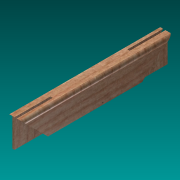
# Autodesk Inventor part: Stretcher-08
Saved by Autodesk Inventor 2013 (Build 170138000, 138)
## iProperties
Created: 2013-08-15
Part Number: Stretcher-08
Material: Wood (Birch)
Document SubType Name: Modeling
Designer: Sawaiz
Density: 1 g/cm^3
Author: Sawaiz
Autodesk Inventor part; units mm, degrees
ref_plane "YZ Plane" through (0, 0, 0) normal (1, 0, 0) x (0, 1, 0)
ref_plane "XZ Plane" through (0, 0, 0) normal (0, 1, 0) x (-1, 0, 0)
ref_plane "XY Plane" through (0, 0, 0) normal (0, 0, 1) x (1, 0, 0)
sketch "Sketch1" plane through (0, 0, 0) normal (1, 0, 0) x (0, 1, 0)
  line L0 (-19.05, 6.858) -> (19.05, 6.858)
  line L1 (19.05, 6.858) -> (19.05, -6.858)
  line L2 (19.05, -6.858) -> (-19.05, -6.858)
  line L3 (-19.05, -6.858) -> (-19.05, 6.858)
  line L4 (-19.05, 6.858) -> (19.05, -6.858) construction
  line L5 (19.05, 6.858) -> (-19.05, -6.858) construction
  arc A0 (19.05, 6.858) -> (10.414, 6.858) centre (14.732, 4.0649) ccw
  arc A1 (10.414, -6.858) -> (19.05, -6.858) centre (14.732, -4.0649) ccw
  line L6 (14.732, 9.2075) -> (14.732, -9.2075)
  point P0 (0, 0)
  dimension "d0" = 38.1
  dimension "d1" = 13.716
  dimension "d6" = 8.636
  dimension "d8" = 8.636
  dimension "d9" = 18.415
  constraints: 14 end point, 6 point on circle, 2 centre point, 2 midpoint, 2 parallel, 2 point on line, 1 equal radius, 1 horizontal, 1 perpendicular
  measures "d0" distance of L1.end L2.end
  measures "d1" distance of L0.end L1.end
  measures "d6" distance of A0.end L0.end
  measures "d8" distance of A1.start L1.end
  measures "d9" distance of L6.start L6.end
extrude "Extrusion1" add sketch "Sketch1" along normal mid plane 203.2
sketch "Sketch3" plane through (-101.6, -19.05, -6.858) normal (0, -1, 0) x (1, 0, 0)
  line L0 (0, 0) -> (203.2, 0) projected
  line L1 (203.2, 13.716) -> (203.2, 0) projected
  line L2 (203.2, 13.716) -> (0, 13.716) projected
  line L3 (0, 0) -> (0, 13.716) projected
  line L4 (203.2, 6.858) -> (154.94, 6.858)
  line L5 (154.94, 6.858) -> (154.94, 3.8)
  line L6 (154.94, 3.8) -> (203.2, 3.8)
  line L7 (203.2, 3.8) -> (203.2, 6.858)
  line L8 (154.94, 6.858) -> (203.2, 6.858)
  line L9 (203.2, 6.858) -> (203.2, 9.916)
  line L10 (0, 9.916) -> (48.26, 9.916)
  line L11 (48.26, 9.916) -> (48.26, 6.858)
  line L12 (48.26, 6.858) -> (0, 6.858)
  line L13 (0, 6.858) -> (0, 9.916)
  point P0 (101.6, 6.858)
  dimension "d14" = 48.26
  dimension "d19" = 3.8
  dimension "d21" = 3.058
  dimension "d22" = 48.26
  dimension "d23" = 3.8
  dimension "d24" = 3.058
  constraints: 20 end point, 4 parallel, 3 horizontal, 3 perpendicular, 2 point on line, 1 midpoint
  measures "d14" distance between parallel lines of L7 L5
  measures "d19" distance between parallel lines of L0 L6
  measures "d21" distance of L4.end L5.end
  measures "d22" distance between parallel lines of L11 L13
  measures "d23" distance between parallel lines of L2 L10
  measures "d24" distance between parallel lines of L12 L10
extrude "Extrusion3" cut sketch "Sketch3" against normal through all contours L3 L10 L11 L12 | L6 L5 L4 L1
ref_plane "Work Plane1" through (-101.6, 10.414, 26.858) normal (0, 0, 1) x (1, 0, 0)
sketch "Sketch4" plane through (-101.6, 10.414, 26.858) normal (0, 0, 1) x (1, 0, 0)
  line L0 (0, 0) -> (203.2, 0) projected
  line L1 (0, -29.464) -> (0, 0) projected
  line L2 (203.2, -29.464) -> (0, -29.464) projected
  line L3 (203.2, 0) -> (203.2, -29.464) projected
  line L4 (0, 0) -> (203.2, 0) projected
  line L5 (203.2, 8.636) -> (203.2, 0) projected
  line L6 (0, 8.636) -> (203.2, 8.636) projected
  line L7 (0, 0) -> (0, 8.636) projected
  line L8 (203.2, 8.636) -> (165.1, -29.464)
  line L9 (0, 8.636) -> (38.1, -29.464)
  line L10 (203.2, 8.636) -> (203.2, -29.464)
  line L11 (165.1, -29.464) -> (203.2, -29.464)
  line L12 (38.1, -29.464) -> (0, -29.464)
  line L13 (0, 8.636) -> (0, -29.464)
  point P0 (101.6, -10.414)
  dimension "d28" = 45
  dimension "d29" = 45
  constraints: 12 end point, 2 collinear, 2 point on line, 1 parallel, 1 perpendicular
  measures "d28" angle of L2 L9
  measures "d29" angle of L2 L8
extrude "Extrusion4" cut sketch "Sketch4" against normal blind 23.8 contours L7 L9 L0 | L0 L9 L2 L1 | L8 L5 L0 | L0 L3 L2 L8
ref_plane "Work Plane2" through (101.6, 10.414, -26.858) normal (0, 0, -1) x (-1, 0, 0)
sketch "Sketch5" plane through (101.6, 10.414, -26.858) normal (0, 0, -1) x (-1, 0, 0)
  line L0 (203.2, 0) -> (0, 0) projected
  line L1 (0, -29.464) -> (0, 0) projected
  line L2 (203.2, -29.464) -> (0, -29.464) projected
  line L3 (203.2, 0) -> (203.2, -29.464) projected
  line L4 (0, 8.636) -> (203.2, 8.636) projected
  line L5 (0, 0) -> (0, 8.636) projected
  line L6 (203.2, 0) -> (0, 0) projected
  line L7 (203.2, 8.636) -> (203.2, 0) projected
  line L8 (0, 8.636) -> (38.1, -29.464)
  line L9 (203.2, 8.636) -> (165.1, -29.464)
  line L10 (165.1, -29.464) -> (203.2, -29.464)
  line L11 (203.2, -29.464) -> (203.2, 8.636)
  line L12 (38.1, -29.464) -> (0, -29.464)
  line L13 (0, -29.464) -> (0, 8.636)
  point P0 (101.6, -10.414)
  dimension "d33" = 45
  dimension "d34" = 45
  constraints: 12 end point, 3 perpendicular, 2 point on line, 1 collinear
  measures "d33" angle of L12 L8
  measures "d34" angle of L2 L9
extrude "Extrusion5" cut sketch "Sketch5" against normal blind 23.8 contours L3 L2 L9 L0 | L0 L9 L7 | L8 L2 L1 L0 | L0 L5 L8
equation "\"d14\" = SlotDepth"
equation "\"d19\" = SlotOffset"
equation "\"d21\" = SlotWidth"
equation "\"d22\" = SlotDepth"
equation "\"d23\" = SlotOffset"
equation "\"d24\" = SlotWidth"
equation "\"d0\" = StretcherHeight"
equation "\"d1\" = StretcherDepth"
equation "\"d6\" = RoundoverDiameter"
equation "\"d8\" = d6"
equation "\"SlotDepth\" = 48.26"
equation "\"SlotOffset\" = 3.8"
equation "\"SlotWidth\" = 3.058"
equation "\"StretcherHeight\" = 38.1"
equation "\"StretcherDepth\" = 13.716"
equation "\"RoundoverDiameter\" = 8.636"
body "Solid2"
